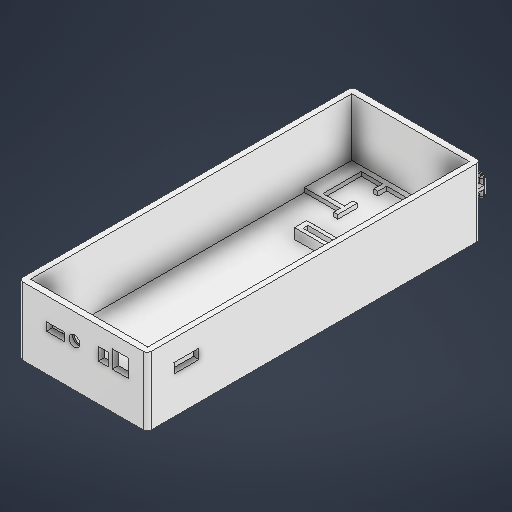
# Autodesk Inventor part: module_command
Saved by Autodesk Inventor 2025.4 (Build 294407000, 407)
## iProperties
Created: 2025-09-05
Part Number: module_command
Material: PC/ABS Plastic
Document SubType Name: Modeling
Designer: sam
Density: 1.1 g/cm^3
Appearance: Smooth - White
Author: sam
Autodesk Inventor part; units mm, degrees
ref_plane "YZ Plane" through (0, 0, 0) normal (1, 0, 0) x (0, 1, 0)
ref_plane "XZ Plane" through (0, 0, 0) normal (0, 1, 0) x (-1, 0, 0)
ref_plane "XY Plane" through (0, 0, 0) normal (0, 0, 1) x (1, 0, 0)
sketch "Sketch1" plane through (0, 0, 0) normal (0, 1, 0) x (-1, 0, 0)
  line L0 (-31.2, -81) -> (31.2, -81)
  line L1 (31.2, -81) -> (31.2, 81)
  line L2 (31.2, 81) -> (-31.2, 81)
  line L3 (-31.2, 81) -> (-31.2, -81)
  line L4 (-31.2, -81) -> (31.2, 81) construction
  line L5 (31.2, -81) -> (-31.2, 81) construction
  point P0 (0, 0)
  dimension "d0" = 62.4
  dimension "d1" = 162
  constraints: 12 end point, 2 midpoint, 2 parallel, 1 horizontal, 1 perpendicular
  measures "d0" distance of L2.end L1.end
  measures "d1" distance of L1.end L0.end
extrude "Extrusion1" add sketch "Sketch1" along normal blind 3
sketch "Sketch2" plane through (0, 3, 0) normal (0, 1, 0) x (1, 0, 0)
  line L0 (-31.2, 81) -> (-31.2, -81) projected
  line L1 (-31.2, -81) -> (31.2, -81) projected
  line L2 (31.2, -81) -> (31.2, 81) projected
  line L3 (31.2, 81) -> (-31.2, 81) projected
  line L4 (31.2, 81) -> (-31.2, 81)
  line L5 (-31.2, 81) -> (-31.2, -81)
  line L6 (-31.2, -81) -> (31.2, -81)
  line L7 (31.2, -81) -> (31.2, 81)
  line L8 (28.5, 78) -> (-28.5, 78)
  line L9 (-28.5, 78) -> (-28.5, -78)
  line L10 (-28.5, -78) -> (28.5, -78)
  line L11 (28.5, -78) -> (28.5, 78)
  point P0 (0, 0)
  dimension "d175" = 2.7
  dimension "d176" = 2.7
  dimension "d177" = 3
  dimension "d178" = 3
  constraints: 16 end point, 4 parallel, 2 horizontal, 2 perpendicular
  measures "d175" distance between parallel lines of L0 L9
  measures "d176" distance between parallel lines of L2 L11
  measures "d177" distance between parallel lines of L1 L10
  measures "d178" distance between parallel lines of L3 L8
extrude "Extrusion2" add sketch "Sketch2" along normal blind 30
fillet "Fillet1" radius 2 4 edges at (31.2, 16.5, 81) (31.2, 16.5, -81) (-31.2, 16.5, 81) (-31.2, 16.5, -81)
sketch "Sketch9" plane through (0, 3, 0) normal (0, 1, 0) x (1, 0, 0)
  line L0 (28.5, 78) -> (-28.5, 78) projected
  line L1 (-28.5, 78) -> (-28.5, -78) projected
  line L2 (-28.5, -78) -> (28.5, -78) projected
  line L3 (28.5, -78) -> (28.5, 78) projected
  line L4 (-28.5, -75.5) -> (28.5, -75.5)
  line L5 (28.5, -75.5) -> (28.5, -73.6)
  line L6 (28.5, -73.6) -> (-28.5, -73.6)
  line L7 (-28.5, -73.6) -> (-28.5, -75.5)
  line L8 (-28.5, 78) -> (-28.5, -78) projected
  line L9 (-28.5, 32.8) -> (28.5, 32.8)
  line L10 (28.5, 32.8) -> (28.5, 34.55)
  line L11 (28.5, 34.55) -> (-28.5, 34.55)
  line L12 (-28.5, 34.55) -> (-28.5, 32.8)
  line L13 (-28.5, 34.55) -> (-11.1, 34.55)
  line L14 (-11.1, 34.55) -> (-11.1, 32.8)
  line L15 (-11.1, 32.8) -> (-28.5, 32.8)
  line L16 (-28.5, 32.8) -> (-28.5, 34.55)
  line L17 (28.5, 38.7) -> (-11.1, 38.7)
  line L18 (-11.1, 38.7) -> (-11.1, 36.95)
  line L19 (-11.1, 36.95) -> (28.5, 36.95)
  line L20 (28.5, 36.95) -> (28.5, 38.7)
  line L21 (-11.1, 36.95) -> (-8.7, 36.95)
  line L22 (-8.7, 36.95) -> (-8.7, 34.55)
  line L23 (-8.7, 34.55) -> (-11.1, 34.55)
  line L24 (-11.1, 34.55) -> (-11.1, 36.95)
  point P0 (0, 0)
  point P1 (28.5, 14.2)
  point P2 (-28.5, 34.55)
  point P3 (-28.5, 32.8)
  point P4 (28.5, 32.8)
  point P5 (-28.5, -73.6)
  point P6 (28.5, -75.5)
  point P7 (-11.1, 34.55)
  point P8 (28.5, 36.95)
  dimension "d79" = 1.9
  dimension "d80" = 2.5
  dimension "d81" = 1.75
  dimension "d82" = 106.4
  dimension "d87" = 17.4
  dimension "d163" = 1.75
  dimension "d164" = 2.4
  dimension "d165" = 17.4
  dimension "d166" = 2.4
  constraints: 40 end point, 10 parallel, 8 point on line, 5 horizontal, 5 perpendicular
  measures "d79" distance of L5.end L4.end
  measures "d80" distance between parallel lines of L2 L4
  measures "d81" distance of L10.end L9.end
  measures "d82" distance between parallel lines of L6 L9
  measures "d87" distance of L14.end L15.end
  measures "d163" distance between parallel lines of L17 L19
  measures "d164" distance between parallel lines of L11 L19
  measures "d165" distance between parallel lines of L8 L18
  measures "d166" distance of L22.end L23.end
extrude "Extrusion9" add sketch "Sketch9" along normal blind 5 contours L3 L19 L18 L17 | L24 L19 L22 L11 | L11 L3 L9 L14 | L6 L3 L4 L1
sketch "Sketch10" plane through (0, 3, 0) normal (0, 1, 0) x (1, 0, 0)
  line L0 (-28.5, -73.6) -> (28.5, -73.6) projected
  line L1 (28.5, -73.6) -> (28.5, 32.8) projected
  line L2 (28.5, 32.8) -> (-11.1, 32.8) projected
  line L3 (-8.7, 34.55) -> (28.5, 34.55) projected
  line L4 (28.5, 34.55) -> (28.5, 36.95) projected
  line L5 (28.5, 78) -> (-28.5, 78) projected
  line L6 (-28.5, 78) -> (-28.5, -73.6) projected
  line L7 (-28.5, 36.7) -> (28.5, 36.7)
  line L8 (-28.5, 69.9) -> (-28.5, 36.7)
  line L9 (-28.5, 36.7) -> (28.5, 36.7)
  line L10 (28.5, 36.7) -> (28.5, 38.7)
  line L11 (28.5, 38.7) -> (-28.5, 38.7)
  line L12 (-28.5, 38.7) -> (-28.5, 36.7)
  line L13 (28.5, 34.55) -> (28.5, 78) projected
  line L14 (-28.5, 38.7) -> (28.5, 38.7)
  line L15 (28.5, 38.7) -> (28.5, 75.6)
  line L16 (28.5, 75.6) -> (-23, 75.6)
  line L17 (-23, 75.6) -> (28.5, 75.6)
  line L18 (28.5, 75.6) -> (28.5, 68)
  line L19 (-23, 73.1) -> (-23, 75.6)
  line L20 (28.5, 38.7) -> (26.5, 38.7)
  line L21 (26.5, 38.7) -> (26.5, 75.6)
  line L22 (26.5, 75.6) -> (28.5, 75.6)
  line L23 (28.5, 75.6) -> (28.5, 38.7)
  line L24 (26.5, 38.7) -> (9.7, 38.7)
  line L25 (9.7, 38.7) -> (9.7, 75.6)
  line L26 (9.7, 75.6) -> (26.5, 75.6)
  line L27 (26.5, 75.6) -> (26.5, 38.7)
  line L28 (9.7, 38.7) -> (7.7, 38.7)
  line L29 (7.7, 38.7) -> (7.7, 75.6)
  line L30 (7.7, 75.6) -> (9.7, 75.6)
  line L31 (9.7, 75.6) -> (9.7, 38.7)
  line L32 (7.7, 38.7) -> (-9.1, 38.7)
  line L33 (-9.1, 38.7) -> (-9.1, 75.6)
  line L34 (-9.1, 75.6) -> (7.7, 75.6)
  line L35 (7.7, 75.6) -> (7.7, 38.7)
  line L36 (-9.1, 38.7) -> (-11.1, 38.7)
  line L37 (-11.1, 38.7) -> (-11.1, 75.6)
  line L38 (-11.1, 75.6) -> (-9.1, 75.6)
  line L39 (-9.1, 75.6) -> (-9.1, 38.7)
  line L40 (-23, 75.6) -> (-21.5, 75.6)
  line L41 (-21.5, 75.6) -> (-21.5, 38.7)
  line L42 (-21.5, 38.7) -> (-23, 38.7)
  line L43 (-23, 38.7) -> (-23, 75.6)
  line L44 (-11.1, 39.2) -> (-11.1, 57)
  line L45 (-11.1, 57) -> (-21.5, 57)
  line L46 (-21.5, 57) -> (-21.5, 38.7)
  line L47 (-11.1, 38.7) -> (28.5, 38.7) projected
  line L48 (28.5, 38.7) -> (28.5, 78) projected
  line L49 (-11.1, 32.8) -> (-11.1, 38.7) projected
  line L50 (28.5, 36.95) -> (-8.7, 36.95) projected
  line L51 (-8.7, 36.95) -> (-8.7, 34.55) projected
  line L52 (28.5, -75.5) -> (-28.5, -75.5) projected
  line L53 (-28.5, -75.5) -> (-28.5, -78) projected
  line L54 (-28.5, -78) -> (28.5, -78) projected
  line L55 (28.5, -78) -> (28.5, -75.5) projected
  line L56 (-11.1, 39.2) -> (-11.1, 36.7)
  line L57 (-11.1, 55) -> (-23, 55)
  line L58 (-11.1, 39.2) -> (-11.1, 32.8)
  line L59 (-11.1, 32.8) -> (-11.1, 32.8)
  line L60 (-11.1, 32.8) -> (-11.1, 39.2)
  line L61 (-23, 55) -> (-28.5, 55)
  line L62 (7.7, 51.8) -> (9.7, 51.8)
  line L63 (9.7, 51.8) -> (9.7, 41.8)
  line L64 (9.7, 41.8) -> (7.7, 41.8)
  line L65 (7.7, 41.8) -> (7.7, 51.8)
  line L66 (-11.1, 41.8) -> (-9.1, 41.8)
  line L67 (-9.1, 41.8) -> (-9.1, 51.8)
  line L68 (-9.1, 51.8) -> (-11.1, 51.8)
  line L69 (-11.1, 51.8) -> (-11.1, 41.8)
  line L70 (-11.1, 71.3) -> (-9.1, 71.3)
  line L71 (-9.1, 71.3) -> (-9.1, 61.3)
  line L72 (-9.1, 61.3) -> (-11.1, 61.3)
  line L73 (-11.1, 61.3) -> (-11.1, 71.3)
  point P0 (0, 0)
  point P1 (28.5, 36.7)
  point P2 (7.7, 38.7)
  point P3 (-9.1, 38.7)
  point P4 (-11.1, 38.7)
  point P5 (-21.5, 38.7)
  point P6 (-21.5, 57)
  point P7 (26.5, 38.7)
  point P8 (9.7, 38.7)
  point P9 (28.2, 37.2)
  point P10 (-11.1, 36.7)
  point P11 (-25.2, 72.6)
  point P12 (-11.1, 75.6)
  point P13 (-11.1, 36.7)
  point P14 (-11.1, 38.7)
  point P15 (-21.5, 75.6)
  point P16 (-25.2, 52)
  point P17 (-11.1, 36.7)
  point P18 (-28.5, 38.7)
  point P19 (28.5, 75.6)
  point P20 (28.5, 38.7)
  point P21 (-11.1, 36.7)
  point P22 (-11.1, 38.7)
  point P23 (-21.5, 55)
  point P24 (-11.1, 38.7)
  point P25 (-10.7, 32.8)
  point P26 (28.5, 38.7)
  point P27 (-11.1, 38.7)
  point P28 (-9.1, 38.7)
  point P29 (-28.5, 55)
  point P30 (7.7, 41.8)
  point P31 (-9.1, 41.8)
  point P32 (-9.1, 51.8)
  point P33 (-11.1, 61.3)
  point P34 (7.7, 51.8)
  point P35 (9.7, 51.8)
  dimension "d90" = 2
  dimension "d91" = 36.9
  dimension "d93" = 2
  dimension "d94" = 16.8
  dimension "d95" = 2
  dimension "d96" = 16.8
  dimension "d97" = 2
  dimension "d98" = 1.5
  dimension "d167" = 2.4
  dimension "d172" = 18.6
  dimension "d173" = 2
  dimension "d174" = 10.4
  dimension "d179" = 10
  dimension "d180" = 10
  dimension "d181" = 3.1
  dimension "d182" = 3.1
  dimension "d183" = 10
  dimension "d184" = 4.3
  constraints: 114 end point, 23 parallel, 21 point on line, 14 perpendicular, 13 horizontal, 1 collinear
  measures "d90" distance of L10.end L9.end
  measures "d91" distance of L15.end L14.end
  measures "d93" distance of L21.end L22.end
  measures "d94" distance of L25.end L26.end
  measures "d95" distance of L29.end L30.end
  measures "d96" distance of L33.end L34.end
  measures "d97" distance of L37.end L38.end
  measures "d98" distance of L41.end L42.end
  measures "d167" distance between parallel lines of L5 L16
  measures "d172" distance between parallel lines of L16 L45
  measures "d173" distance between parallel lines of L45 L57
  measures "d174" distance between parallel lines of L37 L41
  measures "d179" distance of L62.end L63.end
  measures "d180" distance of L67.end L66.end
  measures "d181" distance between parallel lines of L36 L66
  measures "d182" distance between parallel lines of L14 L64
  measures "d183" distance of L70.end L71.end
  measures "d184" distance between parallel lines of L34 L70
extrude "Extrusion10" add sketch "Sketch10" along normal blind 2 contours L6 L5 L13 L16 L19 L43 L61 | L37 L66 L33 L11 | L43 L19 L16 L41 L57 | L41 L45 L37 L57 | L29 L64 L25 L11 | L37 L72 L33 L68 | L11 L21 L16 L13 | L29 L16 L25 L62 | L16 L33 L70 L37
sketch "Sketch11" plane through (-23.2, 5, 81) normal (0, 0, 1) x (1, 0, 0)
  line L0 (-6, 28) -> (52.4, 28) projected
  line L1 (5.5, 13) -> (14.4, 13)
  line L2 (14.4, 13) -> (14.4, 17)
  line L3 (14.4, 17) -> (5.5, 17)
  line L4 (5.5, 17) -> (5.5, 13)
  line L5 (45.4, 13) -> (37.34, 13)
  line L6 (37.34, 13) -> (37.34, 21.6)
  line L7 (37.34, 21.6) -> (45.4, 21.6)
  line L8 (45.4, 21.6) -> (45.4, 13)
  circle A0 centre (19, 15.65) radius 2.65
  line L9 (48.4, 0) -> (48.4, 30) projected
  line L10 (52.4, 28) -> (52.4, -5) projected
  line L11 (-6, -5) -> (-6, 28) projected
  line L12 (-6, -5) -> (52.4, -5) projected
  line L13 (54.4, -5) -> (54.4, 28) projected
  line L14 (-8, 28) -> (-8, -5) projected
  line L15 (30.64, 13) -> (35.34, 13)
  line L16 (35.34, 13) -> (35.34, 19.2)
  line L17 (35.34, 19.2) -> (30.64, 19.2)
  line L18 (30.64, 19.2) -> (30.64, 13)
  point P0 (23.2, -5)
  point P1 (46.4, 0)
  point P2 (0, 0)
  dimension "d110" = 8.9
  dimension "d111" = 4
  dimension "d112" = 8.06
  dimension "d113" = 8.6
  dimension "d114" = 5.3
  dimension "d149" = 9
  dimension "d150" = 13.5
  dimension "d151" = 27
  dimension "d152" = 18
  dimension "d153" = 18
  dimension "d154" = 18
  dimension "d168" = 4.7
  dimension "d169" = 6.2
  dimension "d170" = 2
  dimension "d171" = 18
  constraints: 24 end point, 6 parallel, 3 horizontal, 3 perpendicular, 1 centre point
  measures "d110" distance of L3.end L2.end
  measures "d111" distance of L2.end L1.end
  measures "d112" distance of L6.end L7.end
  measures "d113" distance of L5.end L6.end
  measures "d114" diameter of A0
  measures "d149" distance between parallel lines of L8 L13
  measures "d150" distance between parallel lines of L14 L4
  measures "d151" distance from line of A0.centre L14
  measures "d152" distance between parallel lines of L12 L5
  measures "d153" distance between parallel lines of L12 L1
  measures "d154" distance edge to line of A0 L12
  measures "d168" distance of L17.end L16.end
  measures "d169" distance of L16.end L15.end
  measures "d170" distance between parallel lines of L6 L16
  measures "d171" distance between parallel lines of L12 L15
extrude "Extrusion11" cut sketch "Sketch11" against normal blind 3 contours L4 L3 L2 L1 | L5 L6 L7 L8 | A0 | L18 L17 L16 L15
sketch "Sketch12" plane through (28.5, 3, 78) normal (0, 0, -1) x (-1, 0, 0)
  line L0 (14.36, 23.6) -> (14.36, 15) projected
  line L1 (14.36, 15) -> (6.3, 15) projected
  line L2 (6.3, 15) -> (6.3, 23.6) projected
  line L3 (6.3, 23.6) -> (14.36, 23.6) projected
  line L4 (37.3, 19) -> (46.2, 19) projected
  line L5 (46.2, 19) -> (46.2, 15) projected
  line L6 (46.2, 15) -> (37.3, 15) projected
  line L7 (37.3, 15) -> (37.3, 19) projected
  circle A0 centre (32.7, 17.65) radius 2.65 projected
  line L8 (57, 0) -> (0, 0) projected
  line L9 (57, 0) -> (57, 30) projected
  line L10 (0, 30) -> (57, 30) projected
  line L11 (0, 0) -> (0, 30) projected
  circle A1 centre (32.7, 17.65) radius 3.1
  point P0 (28.5, -3)
  dimension "d128" = 6.2
  constraints: 1 centre point, 1 coincident
  measures "d128" diameter of A1
extrude "Extrusion12" cut sketch "Sketch12" against normal blind 1.2 contours A1
sketch "Sketch13" plane through (23.2, 5, -81) normal (0, 0, -1) x (-1, 0, 0)
  line L0 (-5, 18) -> (51.4, 18)
  line L1 (51.4, 18) -> (51.4, 8.4)
  line L2 (51.4, 8.4) -> (-5, 8.4)
  line L3 (-5, 8.4) -> (-5, 18)
  line L4 (54.4, -5) -> (54.4, 28) projected
  line L5 (-8, 28) -> (-8, -5) projected
  line L6 (-6, -5) -> (52.4, -5) projected
  point P0 (23.2, -5)
  point P1 (51.4, 0)
  point P2 (-5, 0)
  point P3 (54.4, 11.5)
  point P4 (51.4, 13.2)
  dimension "d131" = 9.6
  dimension "d146" = 3
  dimension "d147" = 3
  dimension "d156" = 23
  constraints: 8 end point, 2 parallel, 1 horizontal, 1 midpoint, 1 perpendicular, 3 other
  measures "d131" distance of L0.end L1.end
  measures "d156" distance between parallel lines of L0 L6
extrude "Extrusion13" add sketch "Sketch13" along normal blind 6
sketch "Sketch14" plane through (-28.2, 13.4, -81) normal (-1, 0, 0) x (0, 0, 1)
  line L0 (0, 9.6) -> (0, 0) projected
  line L1 (0, 9.6) -> (-6, 9.6) projected
  line L2 (-6, 0) -> (-6, 9.6) projected
  line L3 (0, 0) -> (-6, 0) projected
  line L4 (0, 9.6) -> (-3.4, 9.6)
  line L5 (-3.4, 9.6) -> (-3.4, 6.6)
  line L6 (-3.4, 6.6) -> (0, 6.6)
  line L7 (0, 6.6) -> (0, 9.6)
  line L8 (0, 0) -> (-3.4, 0)
  line L9 (-3.4, 0) -> (-3.4, 3)
  line L10 (-3.4, 3) -> (0, 3)
  line L11 (0, 3) -> (0, 0)
  point P0 (81, -13.4)
  point P1 (0, 6.6)
  dimension "d137" = 3.4
  dimension "d138" = 3
  dimension "d139" = 3.4
  dimension "d140" = 3
  constraints: 16 end point, 4 parallel, 2 horizontal, 2 perpendicular
  measures "d137" distance of L6.end L5.end
  measures "d138" distance of L5.end L4.end
  measures "d139" distance of L9.end L10.end
  measures "d140" distance of L8.end L9.end
extrude "Extrusion14" cut sketch "Sketch14" against normal up to surface (56.4 mm away) contours L0 L6 L5 L1 | L0 L3 L9 L10
fillet "Fillet5" radius 1 18 edges at (0, 23, -87) (0, 23, -84.4) (0, 13.4, -87) (0, 13.4, -84.4) (-28.2, 16.4, -82.7) (-28.2, 20, -82.7) (28.2, 16.4, -82.7) (28.2, 20, -82.7) (-28.2, 18.2, -87) (-28.2, 21.5, -84.4) (-28.2, 14.9, -84.4) (-28.2, 23, -85.7) (-28.2, 13.4, -85.7) (28.2, 23, -85.7) (28.2, 13.4, -85.7) (28.2, 14.9, -84.4) (28.2, 18.2, -87) (28.2, 21.5, -84.4)
sketch "Sketch15" plane through (31.2, 0, 79) normal (1, 0, 0) x (0, 0, -1)
  line L0 (11, 22.8) -> (23.1, 22.8)
  line L1 (23.1, 22.8) -> (23.1, 18)
  line L2 (23.1, 18) -> (11, 18)
  line L3 (11, 18) -> (11, 22.8)
  line L4 (-2, 33) -> (-2, 0) projected
  line L5 (0, 0) -> (158, 0) projected
  point P0 (79, 0)
  dimension "d157" = 12.1
  dimension "d158" = 4.8
  dimension "d159" = 13
  dimension "d160" = 18
  constraints: 8 end point, 2 parallel, 1 horizontal, 1 perpendicular
  measures "d157" distance of L1.end L2.end
  measures "d158" distance of L0.end L1.end
  measures "d159" distance between parallel lines of L4 L3
  measures "d160" distance between parallel lines of L5 L2
extrude "Extrusion15" cut sketch "Sketch15" against normal blind 3
body "Solid1"
